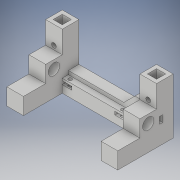
# Autodesk Inventor part: 000.102 - Передняя часть ходовой части
Saved by Autodesk Inventor 2019 (Build 230136000, 136)
## iProperties
Created: 2020-06-05
Part Number: 000.102 - Передняя часть ходовой части
Material: Типовые
Document SubType Name: Modeling
Designer: Петров Иван
Density: 1 g/cm^3
Appearance: По умолчанию
Author: Петров Иван
Autodesk Inventor part; units mm, degrees
ref_plane "YZ Plane" through (0, 0, 0) normal (1, 0, 0) x (0, 1, 0)
ref_plane "XZ Plane" through (0, 0, 0) normal (0, 1, 0) x (-1, 0, 0)
ref_plane "XY Plane" through (0, 0, 0) normal (0, 0, 1) x (1, 0, 0)
sketch "Эскиз1" plane through (0, 0, 0) normal (0, 1, 0) x (-1, 0, 0)
  line L0 (-50, 0) -> (50, 0)
  line L1 (50, 0) -> (50, -50)
  line L2 (50, -50) -> (-50, -50)
  line L3 (-50, -50) -> (-50, 0)
  point P0 (0, 0)
  dimension "d0" = 100
  dimension "d1" = 50
  dimension "d2" = 50
  dimension "d3" = 0
  constraints: 8 end point, 2 parallel, 1 horizontal, 1 perpendicular
  measures "d0" distance of L1.end L2.end
  measures "d1" distance of L0.end L1.end
  measures "d2" distance from line of point (0, 0) L1
  measures "d3" distance from line of point (0, 0) L0
extrude "Выдавливание1" add sketch "Эскиз1" along normal blind 50
sketch "Эскиз2" plane through (0, 50, 0) normal (0, 1, 0) x (1, 0, 0)
  line L0 (-50, 0) -> (50, 0) projected
  line L1 (-35, 0) -> (35, 0)
  line L2 (35, 0) -> (35, 35)
  line L3 (35, 35) -> (-35, 35)
  line L4 (-35, 35) -> (-35, 0)
  line L5 (50, 0) -> (50, 50) projected
  line L6 (-50, 50) -> (-50, 0) projected
  line L7 (50, 50) -> (-50, 50) projected
  dimension "d9" = 15
  dimension "d10" = 15
  dimension "d11" = 15
  constraints: 8 end point, 2 parallel, 1 horizontal, 1 perpendicular, 1 point on line
  measures "d9" distance between parallel lines of L5 L2
  measures "d10" distance between parallel lines of L4 L6
  measures "d11" distance between parallel lines of L7 L3
extrude "Выдавливание2" cut sketch "Эскиз2" against normal through all contours L4 L3 L2 L0
sketch "Эскиз3" plane through (0, 50, 0) normal (0, 1, 0) x (1, 0, 0)
  line L0 (35, 35) -> (12.5, 35)
  line L1 (35, 35) -> (35, 0)
  line L2 (35, 0) -> (50, 0)
  line L3 (50, 0) -> (50, 35)
  line L4 (50, 35) -> (35, 35)
  line L5 (-35, 35) -> (-35, 0)
  line L6 (-50, 50) -> (-50, 0)
  line L7 (-35, 0) -> (-35, 35)
  line L8 (-35, 35) -> (-50, 35)
  line L9 (-50, 35) -> (-50, 0)
  line L10 (-50, 0) -> (-35, 0)
  line L11 (-50, 35) -> (-50, 20)
  line L12 (-50, 20) -> (-35, 20)
  line L13 (-35, 20) -> (-35, 35)
  line L14 (-35, 35) -> (-50, 35)
  line L15 (50, 0) -> (50, 50)
  line L16 (35, 35) -> (35, 20)
  line L17 (35, 20) -> (50, 20)
  line L18 (50, 20) -> (50, 35)
  line L19 (50, 35) -> (35, 35)
  point P0 (0, 0)
  point P1 (0, 0)
  dimension "d14" = 15
  constraints: 40 end point, 8 parallel, 5 point on line, 4 perpendicular
  measures "d14" distance of L13.end L12.end
extrude "Выдавливание3" cut sketch "Эскиз3" against normal blind 35 contours L17 L3 L2 L1 | L5 L10 L6 L12
sketch "Эскиз4" plane through (0, 50, 0) normal (0, 1, 0) x (1, 0, 0)
  line L0 (35, 35) -> (12.5, 35)
  line L1 (35, 35) -> (35, 0)
  line L2 (35, 0) -> (50, 0)
  line L3 (50, 0) -> (50, 35)
  line L4 (50, 35) -> (35, 35)
  line L5 (-35, 35) -> (-35, 0)
  line L6 (-50, 50) -> (-50, 0)
  line L7 (-35, 0) -> (-35, 35)
  line L8 (-35, 35) -> (-50, 35)
  line L9 (-50, 35) -> (-50, 0)
  line L10 (-50, 0) -> (-35, 0)
  line L11 (-50, 35) -> (-50, 20)
  line L12 (-50, 20) -> (-35, 20)
  line L13 (-35, 20) -> (-35, 35)
  line L14 (-35, 35) -> (-50, 35)
  line L15 (50, 0) -> (50, 50)
  line L16 (35, 35) -> (35, 20)
  line L17 (35, 20) -> (50, 20)
  line L18 (50, 20) -> (50, 35)
  line L19 (50, 35) -> (35, 35)
  point P0 (0, 0)
  point P1 (0, 0)
  point P2 (0, 0)
  dimension "d17" = 15
  constraints: 40 end point, 8 parallel, 5 point on line, 4 perpendicular
  measures "d17" distance of L13.end L12.end
extrude "Выдавливание4" cut sketch "Эскиз4" against normal blind 20 contours L4 L3 L17 L1 | L5 L12 L6 L8
sketch "Эскиз5" plane through (0, 50, 0) normal (0, 1, 0) x (1, 0, 0)
  line L0 (-35, 35) -> (-35, 0) projected
  line L1 (-50, 50) -> (50, 50) projected
  line L2 (-35, 35) -> (35, 35)
  line L3 (35, 35) -> (35, 50)
  line L4 (35, 50) -> (-35, 50)
  line L5 (-35, 50) -> (-35, 35)
  line L6 (-50, 35) -> (50, 35) projected
  point P0 (0, 0)
  dimension "d20" = 70
  constraints: 8 end point, 2 parallel, 2 point on line, 1 horizontal, 1 perpendicular
  measures "d20" distance of L4.end L3.end
extrude "Выдавливание5" cut sketch "Эскиз5" against normal up to surface (35 mm away)
sketch "Эскиз6" plane through (50, 0, 0) normal (1, 0, 0) x (0, 0, -1)
  circle A0 centre (27.5, 22.5) radius 5.1
  line L0 (35, 30) -> (20, 30) projected
  line L1 (20, 30) -> (20, 15) projected
  point P0 (0, 0)
  dimension "d23" = 10.2
  dimension "d24" = 7.5
  dimension "d25" = 7.5
  constraints: 1 centre point
  measures "d23" diameter of A0
  measures "d24" distance from line of L0 A0.centre
  measures "d25" distance from line of L1 A0.centre
extrude "Выдавливание6" cut sketch "Эскиз6" against normal blind 112.25
sketch "Эскиз7" plane through (-35, 15, -50) normal (0, 1, 0) x (1, 0, 0)
  line L0 (70, -50) -> (70, -15) projected
  line L1 (0, 0) -> (70, 0) projected
  line L2 (70, -15) -> (60, -15)
  line L3 (60, -15) -> (60, 0)
  line L4 (60, 0) -> (70, 0)
  line L5 (70, 0) -> (70, -15)
  point P0 (35, -50)
  dimension "d28" = 10
  constraints: 8 end point, 2 parallel, 1 horizontal, 1 perpendicular, 1 point on line
  measures "d28" distance of L3.end L4.end
extrude "Выдавливание7" add sketch "Эскиз7" along normal blind 10
sketch "Эскиз8" plane through (50, 0, -50) normal (0, 0, -1) x (-1, 0, 0)
  line L0 (25, 15) -> (25, 25) projected
  line L1 (25, 20) -> (0, 20)
  line L2 (0, 0) -> (0, 50) projected
  line L3 (0, 15) -> (0, 25)
  line L4 (0, 20) -> (25, 20)
  line L5 (25, 15) -> (25, 25)
  circle A0 centre (5, 20) radius 2.1
  circle A1 centre (20, 20) radius 2.1
  point P0 (50, 0)
  point P1 (50, 0)
  dimension "d31" = 4.2
  dimension "d32" = 4.2
  dimension "d33" = 5
  dimension "d34" = 5
  constraints: 8 end point, 4 midpoint, 3 point on line, 2 centre point, 1 horizontal
  measures "d31" diameter of A0
  measures "d32" diameter of A1
  measures "d33" distance from line of L5 A1.centre
  measures "d34" distance from line of L3 A0.centre
sketch "Эскиз9" plane through (-35, 25, -50) normal (0, 1, 0) x (1, 0, 0)
  line L0 (60, 0) -> (60, -15) projected
  line L1 (60, -15) -> (70, -15)
  line L2 (70, -15) -> (70, -9.5)
  line L3 (70, -9.5) -> (60, -9.5)
  line L4 (60, -9.5) -> (60, -15)
  point P0 (35, -50)
  dimension "d35" = 10
  dimension "d36" = 5.5
  constraints: 8 end point, 2 parallel, 1 horizontal, 1 perpendicular
  measures "d35" distance of L3.end L2.end
  measures "d36" distance of L2.end L1.end
extrude "Выдавливание8" cut sketch "Эскиз9" against normal up to surface (10 mm away)
extrude "Выдавливание9" cut sketch "Эскиз8" against normal blind 12
sketch "Эскиз10" plane through (35, 50, -50) normal (-1, 0, 0) x (0, 0, 1)
  line L0 (15, -35) -> (9.5, -35) projected
  line L1 (9.5, -25) -> (9.5, -35) projected
  line L2 (9.5, -27.9) -> (9.5, -32.1) projected
  line L3 (0, -32.1) -> (0, -27.9) projected
  line L4 (0, -32.1) -> (9.5, -32.1) projected
  line L5 (0, -27.9) -> (9.5, -27.9) projected
  line L6 (9.5, -27.9) -> (9.5, -32.1) projected
  line L7 (9.5, -30) -> (11, -30)
  line L8 (12.5, -33) -> (9.5, -33)
  line L9 (9.5, -33) -> (9.5, -27)
  line L10 (9.5, -27) -> (12.5, -27)
  line L11 (12.5, -27) -> (12.5, -33)
  line L12 (12.5, -33) -> (9.5, -27) construction
  line L13 (9.5, -33) -> (12.5, -27) construction
  point P0 (50, -50)
  dimension "d45" = 1.5
  dimension "d46" = 3
  dimension "d47" = 6
  constraints: 14 end point, 3 midpoint, 2 horizontal, 2 parallel, 1 perpendicular
  measures "d45" distance of L7.start L7.end
  measures "d46" distance of L9.end L10.end
  measures "d47" distance of L8.end L9.end
extrude "Выдавливание10" cut sketch "Эскиз10" against normal blind 26.5 contours L10 L11 L8 L1
sketch "Эскиз11" plane through (35, 50, -50) normal (-1, 0, 0) x (0, 0, 1)
  line L0 (9.5, -33) -> (12.5, -33) projected
  line L1 (15, -35) -> (9.5, -35) projected
  line L2 (9.5, -33) -> (15, -33)
  line L3 (15, -33) -> (15, -35)
  line L4 (15, -35) -> (9.5, -35)
  line L5 (9.5, -35) -> (9.5, -33)
  point P0 (50, -50)
  constraints: 8 end point, 2 parallel, 1 horizontal, 1 perpendicular
extrude "Выдавливание11" add sketch "Эскиз11" along normal blind 8
chamfer "Фаска1" distance 10 angle 45 1 edges at (25, 15, -45.25)
sketch "Эскиз12" plane through (-35, 25, -50) normal (0, 1, 0) x (1, 0, 0)
  line L0 (50, 0) -> (50, -9.5)
  line L1 (50, -4.75) -> (60, -4.75)
  line L2 (60, -9.5) -> (60, 0)
  line L3 (60, -4.75) -> (60, -3.24)
  line L4 (50, -4.75) -> (50, -6.26)
  line L5 (60, -3.24) -> (60, -6.26)
  line L6 (60, -6.26) -> (50, -6.26)
  line L7 (50, -6.26) -> (50, -3.24)
  line L8 (50, -3.24) -> (60, -3.24)
  line L9 (60, 0) -> (60, -9.5) projected
  point P0 (35, -50)
  point P1 (0, 0)
  point P2 (60, -4.75)
  dimension "d55" = 1.51
  dimension "d56" = 1.51
  constraints: 18 end point, 3 midpoint, 2 parallel, 2 point on line, 1 coincident, 1 perpendicular
  measures "d55" distance of L1.end L3.end
  measures "d56" distance of L4.end L1.start
extrude "Выдавливание12" cut sketch "Эскиз12" against normal up to surface (10 mm away)
sketch "Эскиз13" plane through (-35, 15, -35) normal (0, 1, 0) x (1, 0, 0)
  line L0 (62, 0) -> (62, 5.5) projected
  line L1 (0, 15) -> (0, 0) projected
  line L2 (62, 5.5) -> (0, 5.5)
  line L3 (0, 5.5) -> (0, 0)
  line L4 (0, 0) -> (62, 0)
  line L5 (62, 0) -> (62, 5.5)
  point P0 (35, -35)
  constraints: 8 end point, 2 parallel, 1 horizontal, 1 perpendicular
extrude "Выдавливание13" cut sketch "Эскиз13" against normal blind 3.3
sketch "Эскиз14" plane through (-35, 0, -35) normal (0, 0, 1) x (1, 0, 0)
  line L0 (0, 0) -> (0, 15)
  line L1 (70, 15) -> (70, 0)
  line L2 (0, 9.7) -> (70, 9.7)
  line L3 (70, 9.7) -> (70, 6.7)
  line L4 (70, 6.7) -> (0, 6.7)
  line L5 (0, 6.7) -> (0, 9.7)
  line L6 (22.5, 11.7) -> (0, 11.7)
  line L7 (22.5, 9.7) -> (47.5, 9.7)
  line L8 (47.5, 9.7) -> (47.5, 6.7)
  line L9 (47.5, 6.7) -> (22.5, 6.7)
  line L10 (8.75, 6.7) -> (13.75, 6.7)
  line L11 (13.75, 9.7) -> (8.75, 9.7)
  line L12 (8.75, 9.7) -> (8.75, 6.7)
  line L13 (47.5, 9.7) -> (56.25, 9.7)
  line L14 (56.25, 9.7) -> (56.25, 6.7)
  line L15 (56.25, 6.7) -> (47.5, 6.7)
  line L16 (47.5, 6.7) -> (47.5, 9.7)
  line L17 (8.75, 9.7) -> (8.75, 6.7)
  line L18 (8.75, 9.7) -> (8.75, 6.7)
  line L19 (8.75, 9.7) -> (0, 9.7)
  line L20 (0, 9.7) -> (0, 6.7)
  line L21 (0, 6.7) -> (8.75, 6.7)
  line L22 (8.75, 6.7) -> (8.75, 9.7)
  point P0 (35, 0)
  point P1 (35, 0)
  dimension "d61" = 3
  dimension "d62" = 5
  dimension "d74" = 8.75
  constraints: 46 end point, 10 equal length, 6 point on line, 5 horizontal, 4 perpendicular
  measures "d61" distance between parallel lines of L2 L4
  measures "d62" distance between parallel lines of L6 L4
  measures "d74" distance of L14.end L15.end
extrude "Выдавливание14" cut sketch "Эскиз14" against normal blind 5.6 contours L0 L2 L12 L4 | L8 L2 L14 L4
ref_plane "РабПлоскость1" through (0, 0, -50) normal (1, 0, 0) x (0, 0, -1)
sketch "Эскиз15" plane through (-35, 11.7, -35) normal (0, 1, 0) x (1, 0, 0)
  line L0 (56.25, 5.6) -> (56.25, 0)
  line L1 (56.25, 5.6) -> (47.5, 5.6)
  line L2 (47.5, 0) -> (47.5, 5.6)
  line L3 (56.25, 0) -> (47.5, 0)
  line L4 (8.75, 5.6) -> (8.75, 0)
  line L5 (8.75, 5.6) -> (0, 5.6)
  line L6 (0, 0) -> (0, 5.6)
  line L7 (8.75, 0) -> (0, 0)
  circle A0 centre (4.375, 2.75) radius 1.6
  circle A1 centre (51.875, 2.75) radius 1.6
  line L8 (56.25, 0) -> (56.25, 5.6) projected
  line L9 (47.5, 0) -> (47.5, 5.6) projected
  point P0 (35, -35)
  dimension "d66" = 3.2
  dimension "d67" = 3.2
  dimension "d68" = 2.75
  dimension "d69" = 2.75
  dimension "d70" = 4.375
  dimension "d71" = 4.375
  constraints: 16 end point, 2 centre point
  measures "d66" diameter of A0
  measures "d67" diameter of A1
  measures "d68" distance from line of L3 A1.centre
  measures "d69" distance from line of L7 A0.centre
  measures "d70" distance from line of L2 A1.centre
  measures "d71" distance from line of L6 A0.centre
extrude "Выдавливание15" cut sketch "Эскиз15" against normal blind 5.6 contours A0 | A1
sketch "Эскиз16" plane through (0, 50, 0) normal (0, 1, 0) x (1, 0, 0)
  line L0 (35, 35) -> (50, 35)
  line L1 (35, 50) -> (35, 35)
  line L2 (38.4, 46.6) -> (46.6, 46.6)
  line L3 (46.6, 46.6) -> (46.6, 38.4)
  line L4 (46.6, 38.4) -> (38.4, 38.4)
  line L5 (38.4, 38.4) -> (38.4, 46.6)
  line L6 (38.4, 46.6) -> (46.6, 38.4) construction
  line L7 (46.6, 46.6) -> (38.4, 38.4) construction
  point P0 (0, 0)
  point P1 (0, 0)
  point P2 (42.5, 35)
  point P3 (35, 42.5)
  point P4 (42.5, 42.5)
  dimension "d75" = 8.2
  dimension "d76" = 8.2
  dimension "d77" = 7.5
  dimension "d78" = 7.5
  constraints: 16 end point, 4 midpoint, 2 parallel, 1 horizontal, 1 perpendicular
  measures "d75" distance of L3.end L4.end
  measures "d76" distance of L2.end L3.end
  measures "d77" distance of point (42.5, 35) point (42.5, 42.5)
  measures "d78" distance of point (35, 42.5) point (42.5, 42.5)
extrude "Выдавливание16" cut sketch "Эскиз16" against normal up to surface (20 mm away)
sketch "Эскиз17" plane through (76.1392, -7.1361, -50) normal (0, 0, -1) x (-1, 0, 0)
  line L0 (111.1392, 57.1361) -> (126.1392, 57.1361)
  line L1 (118.6392, 57.1361) -> (118.6392, 40.7361)
  circle A0 centre (118.6392, 40.7361) radius 2.1
  line L2 (111.1392, 37.1361) -> (111.1392, 57.1361) projected
  point P0 (50, 0)
  dimension "d82" = 16.4
  dimension "d81" = 4.2
  constraints: 4 end point, 1 centre point, 1 coincident, 1 midpoint, 1 vertical
  measures "d82" distance of L1.start L1.end
  measures "d81" diameter of A0
extrude "Выдавливание17" cut sketch "Эскиз17" against normal blind 18.5
mirror "Зеркальное отражение1" about plane through (0, 0, -50) normal (1, 0, 0) of "Выдавливание16", "Выдавливание17"
equation "\"d9\" = d10"
equation "\"d32\" = d31"
equation "\"d33\" = d34"
equation "\"d56\" = d55"
equation "\"d66\" = d67"
equation "\"d69\" = d68"
equation "\"d71\" = d70"
equation "\"d75\" = d76"
